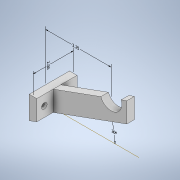
# Autodesk Inventor part: PipeSupport-3_25-020
Saved by Autodesk Inventor 2021.1 (Build 251245010, 245A)
## iProperties
Created: 2020-09-15
Part Number: PipeSupport-3_25-020
Material: Generic
Document SubType Name: Modeling
Designer: robst
Density: 1 g/cm^3
Appearance: Default
Author: robst
Autodesk Inventor part; units mm, degrees
ref_plane "YZ Plane" through (0, 0, 0) normal (1, 0, 0) x (0, 1, 0)
ref_plane "XZ Plane" through (0, 0, 0) normal (0, 1, 0) x (-1, 0, 0)
ref_plane "XY Plane" through (0, 0, 0) normal (0, 0, 1) x (1, 0, 0)
sketch "Sketch5" plane through (0, 0, 0) normal (0, 0, 1) x (1, 0, 0)
  line L0 (0, 0) -> (9.525, 0)
  line L1 (9.525, 0) -> (9.525, 25.4)
  line L2 (9.525, 25.4) -> (0, 25.4)
  line L3 (0, 25.4) -> (0, 0)
  dimension "d21" = 25.4
  dimension "d22" = 9.525
  constraints: 8 end point, 2 parallel, 1 horizontal, 1 perpendicular
  measures "d21" distance from line of L2 L0.start
  measures "d22" distance from line of L1 L0.start
extrude "Extrusion3" add sketch "Sketch5" against normal mid plane 50.8
sketch "Sketch6" plane through (0, 0, 0) normal (0, 0, 1) x (1, 0, 0)
  line L0 (9.525, 25.4) -> (9.525, 0) projected
  line L1 (0, 25.4) -> (9.525, 25.4) projected
  line L2 (9.525, 0) -> (0, 0) projected
  line L3 (0, 0) -> (0, 25.4) projected
  line L4 (9.525, 0) -> (102.5525, 33.8592)
  line L5 (9.525, 0) -> (108.5228, 0) construction
  line L6 (102.5525, 59.2592) -> (102.5525, 33.8592)
  arc A0 (69.7208, 47.3095) -> (95.3792, 56.6484) centre (82.55, 51.9789) ccw
  line L7 (9.525, 25.4) -> (69.7208, 47.3095)
  line L8 (95.3792, 56.6484) -> (102.5525, 59.2592)
  dimension "d25" = 20
  dimension "d26" = 27.305
  dimension "d29" = 6.35
  dimension "d30" = 82.55
  dimension "d33" = 0
  constraints: 10 end point, 2 parallel, 2 point on circle, 1 centre point, 1 collinear, 1 equal length, 1 horizontal, 1 vertical
  measures "d25" angle of L5 L4
  measures "d26" diameter of A0
  measures "d29" distance edge to line of A0 L6
  measures "d30" distance from line of A0.centre L3
  measures "d33" distance from line of L7 A0.centre
extrude "Extrusion4" add sketch "Sketch6" along normal mid plane 9.525 contours L7 A0 L8 L6 L4 L0
sketch "Sketch7" plane through (9.525, 0, 25.4) normal (1, 0, 0) x (0, 0, -1)
  line L0 (50.8, 25.4) -> (0, 25.4) construction
  line L1 (9.525, 25.4) -> (9.525, 0) construction
  line L2 (41.275, 25.4) -> (41.275, 0) construction
  line L3 (0, 0) -> (0, 25.4) construction
  line L4 (50.8, 25.4) -> (50.8, 0) construction
  line L5 (0, 0) -> (20.6375, 0) projected
  line L6 (30.1625, 0) -> (50.8, 0) projected
  point P0 (25.4, 0)
  point P1 (9.525, 12.7)
  point P2 (41.275, 12.7)
  dimension "d34" = 9.525
  dimension "d35" = 9.525
  constraints: 4 end point, 2 midpoint, 2 point on line, 2 vertical
  measures "d34" distance between parallel lines of L1 L3
  measures "d35" distance between parallel lines of L2 L4
sketch "Sketch8" plane through (0, 0, 0) normal (0, 0, 1) x (1, 0, 0)
  line L0 (0, 0) -> (0, 25.4) projected
  line L1 (9.525, 0) -> (0, 0) projected
  line L2 (102.5525, 33.8592) -> (9.525, 0) projected
  line L3 (0, 0) -> (9.525, 0)
  line L4 (0, -3.4668) -> (9.525, 0)
  line L5 (0, 0) -> (0, -3.4668)
  constraints: 6 end point, 2 collinear, 1 vertical
extrude "Extrusion5" add sketch "Sketch8" along normal mid plane 50.8
hole "Hole3" at (9.525, 12.7, 15.875) at (9.525, 12.7, -15.875) direction (-1, 0, 0) diameter 3.81 end through all countersink diameter 7.0866 countersink angle 82 clearance for "Flat Head Machine Screw (82)" size "#6" standard "Ansi Unified Screw Threads"
equation "\"d21\" = supportHeight"
equation "\"d22\" = supportWidth"
equation "\"d23\" = totalScrewHoldWidth"
equation "\"d25\" = supportAngle"
equation "\"d26\" = pipeDiameter"
equation "\"d30\" = distanceFromWallToPipeCenter"
equation "\"d31\" = supportWidth"
equation "\"d47\" = totalScrewHoldWidth"
equation "\"pipeDiameter\" = 27.305"
equation "\"distanceFromWallToPipeCenter\" = 82.55"
equation "\"supportHeight\" = 25.4"
equation "\"supportWidth\" = 9.525"
equation "\"screwHoldDepth\" = 6.35"
equation "\"totalScrewHoldWidth\" = 50.8"
equation "\"screwPositionFromTop\" = 6.35"
equation "\"supportAngle\" = 20deg"
body "Solid1"
body "Solid2"
